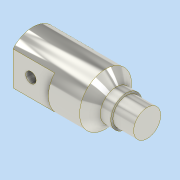
# Autodesk Inventor part: McCrea_krk_walle
Saved by Autodesk Inventor 2021 (Build 250183000, 183)
## iProperties
Created: 2022-01-10
Part Number: McCrea_krk_walle
Material: Generic
Document SubType Name: Modeling
Designer: student
Density: 1 g/cm^3
Appearance: Silver
Author: student
Autodesk Inventor part; units mm, degrees
ref_plane "YZ Plane" through (0, 0, 0) normal (1, 0, 0) x (0, 1, 0)
ref_plane "XZ Plane" through (0, 0, 0) normal (0, 1, 0) x (-1, 0, 0)
sketch "Sketch1" plane through (0, 0, 0) normal (0, 0, 1) x (1, 0, 0)
  line L0 (0, 0) -> (55, 0)
  line L1 (0, 0) -> (0, 12.5)
  line L2 (0, 12.5) -> (40, 12.5)
  line L3 (40, 12.5) -> (40, 7.5)
  line L4 (40, 7.5) -> (45, 7.5)
  line L5 (45, 7.5) -> (45, 6.5)
  line L6 (45, 6.5) -> (55, 6.5)
  line L7 (55, 6.5) -> (55, 0)
  dimension "d5" = 25
  dimension "d6" = 5
  dimension "d7" = 15
  dimension "d8" = 13
  dimension "d9" = 10
  dimension "d10" = 40
  constraints: 16 end point, 4 perpendicular, 2 vertical, 1 horizontal, 1 parallel
  measures "d5" diameter of L2 L0
  measures "d6" distance of L3.end L4.end
  measures "d7" diameter of L4 L0
  measures "d8" diameter of L6 L0
  measures "d9" distance of L5.end L6.end
  measures "d10" distance of L1.end L2.end
revolve "Revolution1" add sketch "Sketch1" angle 360 about axis through (0, 0, 0) along (1, 0, 0)
chamfer "Chamfer1" distance 5 angle 45 1 edges at (40, -12.5, 0)
ref_plane "Work Plane1" through (20, 0, 12.5) normal (0, 0, 1) x (1, 0, 0)
sketch "Sketch2" plane through (20, 0, 12.5) normal (0, 0, 1) x (1, 0, 0)
  line L0 (-20, -12.5) -> (-20, 12.5) projected
  line L1 (0, 10) -> (-20, 10)
  line L2 (-20, 10) -> (-20, -10)
  line L3 (-20, -10) -> (0, -10)
  line L4 (0, -10) -> (0, 10)
  line L5 (-20, -12.5) -> (-20, 12.5) projected
  line L6 (15, -12.5) -> (15, 12.5) projected
  line L7 (-20, -12.5) -> (15, -12.5) projected
  line L8 (-20, 12.5) -> (15, 12.5) projected
  line L9 (15, -12.5) -> (15, 12.5) projected
  point P0 (-20, 0)
  point P1 (-20, 10)
  dimension "d11" = 20
  dimension "d14" = 20
  dimension "d15" = 2.5
  dimension "d16" = 2.5
  dimension "d19" = 25
  constraints: 8 end point, 2 parallel, 1 horizontal, 1 perpendicular, 1 point on line
  measures "d11" distance of L1.start L1.end
  measures "d14" distance of L3.end L1.start
  measures "d15" distance between parallel lines of L8 L1
  measures "d16" distance between parallel lines of L7 L3
  measures "d19" distance of L6.start L6.end
extrude "Extrusion1" cut sketch "Sketch2" against normal blind 3 contours L0 L1 L4 L3
mirror "Mirror1" about plane through (0, 0, 0) normal (0, 0, 1) of "Extrusion1"
sketch "Sketch3" plane through (20, 0, 9.5) normal (0, 0, 1) x (1, 0, 0)
  point P0 (-20, 0)
  point P1 (-11.3903, 0.5397)
hole "Hole1" at (8.6097, 0.5397, 9.5) direction (0, 0, -1) diameter 5 end through all
equation "\"d15\" = -0.5 * d14 + 0.5 * d19"
body "Solid1"
